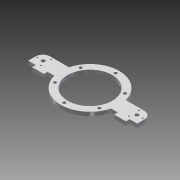
# Autodesk Inventor part: middle plate2
Saved by Autodesk Inventor 2015 (Build 190159000, 159)
## iProperties
Created: 2015-02-28
Part Number: middle plate2
Material: Generic
Document SubType Name: Modeling
Designer: Qiuyang
Density: 1 g/cm^3
Appearance: Default
Author: Qiuyang
Autodesk Inventor part; units mm, degrees
ref_plane "YZ Plane" through (0, 0, 0) normal (1, 0, 0) x (0, 1, 0)
ref_plane "XZ Plane" through (0, 0, 0) normal (0, 1, 0) x (-1, 0, 0)
ref_plane "XY Plane" through (0, 0, 0) normal (0, 0, 1) x (1, 0, 0)
sketch "Sketch4" plane through (0, 0, 0) normal (0, 1, 0) x (-1, 0, 0)
  circle A0 centre (0, 0) radius 38.735
  circle A1 centre (0, 0) radius 50.8
  dimension "d9" = 77.47
  dimension "d10" = 101.6
  constraints: 2 centre point, 2 coincident
  measures "d9" diameter of A0
  measures "d10" diameter of A1
extrude "Extrusion2" add sketch "Sketch4" along normal blind 6.35
sketch "Sketch5" plane through (0, 6.35, 0) normal (0, 1, 0) x (1, 0, 0)
  circle A0 centre (0, -44.45) radius 2.667
  circle A1 centre (38.4948, -22.225) radius 2.667
  circle A2 centre (38.4948, 22.225) radius 2.667
  circle A3 centre (0, 44.45) radius 2.667
  circle A4 centre (-38.4948, 22.225) radius 2.667
  circle A5 centre (-38.4948, -22.225) radius 2.667
  point P0 (0, 0)
  dimension "d13" = 5.334
  dimension "d16" = 360
  constraints: 6 centre point, 13 other
  measures "d13" diameter of A0
extrude "Extrusion3" cut sketch "Sketch5" against normal blind 6.35
sketch "Sketch7" plane through (0, 6.35, 0) normal (0, 1, 0) x (1, 0, 0)
  line L0 (50.8, 12.7) -> (81.788, 12.7)
  line L1 (81.788, 12.7) -> (81.788, -12.7)
  line L2 (81.788, -12.7) -> (50.8, -12.7)
  line L3 (50.8, -12.7) -> (50.8, 12.7)
  line L4 (-50.8, 12.7) -> (-81.788, 12.7)
  line L5 (-81.788, 12.7) -> (-81.788, -12.7)
  line L6 (-81.788, -12.7) -> (-50.8, -12.7)
  line L7 (-50.8, -12.7) -> (-50.8, 12.7)
  point P0 (0, 0)
  dimension "d50" = 30.988
  dimension "d51" = 25.4
  dimension "d52" = 30.988
  constraints: 16 end point, 4 parallel, 2 horizontal, 2 perpendicular, 2 point on line
  measures "d50" distance of L1.end L2.end
  measures "d51" distance of L0.end L1.end
  measures "d52" distance of L6.end L5.end
extrude "Extrusion4" add sketch "Sketch7" against normal blind 6.35
sketch "Sketch8" plane through (0, 6.35, 0) normal (0, 1, 0) x (1, 0, 0)
  line L0 (-123.5202, 12.7) -> (-50.8, 12.7) projected
  line L1 (-60.9386, 12.7) -> (-45.3133, 12.7)
  line L2 (-45.3133, 12.7) -> (-45.3133, -12.7)
  line L3 (-45.3133, -12.7) -> (-60.9386, -12.7)
  line L4 (-60.9386, -12.7) -> (-60.9386, 12.7)
  line L5 (57.1886, 12.7) -> (43.7508, 12.7)
  line L6 (43.7508, 12.7) -> (43.7508, -12.7)
  line L7 (43.7508, -12.7) -> (57.1886, -12.7)
  line L8 (57.1886, -12.7) -> (57.1886, 12.7)
  point P0 (0, 0)
  constraints: 16 end point, 4 parallel, 3 point on line, 2 horizontal, 2 perpendicular
extrude "Extrusion5" add sketch "Sketch8" against normal blind 6.35
sketch "Sketch9" plane through (0, 6.35, 0) normal (0, 1, 0) x (1, 0, 0)
  line L0 (111.76, 12.7) -> (111.76, -12.7) projected
  line L1 (81.788, 12.7) -> (81.788, -12.7) projected
  circle A0 centre (81.788, 0) radius 12.7
  line L2 (-81.788, 12.7) -> (-81.788, -12.7) projected
  circle A1 centre (-81.788, 0) radius 12.7
  point P0 (0, 0)
  point P1 (-111.7602, 0)
  point P2 (-111.76, -12.7)
  constraints: 2 midpoint, 2 vertical alignment, 4 other
extrude "Extrusion6" add sketch "Sketch9" against normal blind 6.35
sketch "Sketch10" plane through (0, 6.35, 0) normal (0, 1, 0) x (1, 0, 0)
  circle A0 centre (81.28, 0) radius 3.175
  circle A1 centre (91.3638, 0) radius 1.27
  circle A2 centre (76.2381, 8.7328) radius 1.27
  circle A3 centre (76.2381, -8.7328) radius 1.27
  circle A4 centre (-81.28, 0) radius 3.175
  circle A5 centre (-91.3638, 0) radius 1.27
  circle A6 centre (-76.2381, -8.7328) radius 1.27
  circle A7 centre (-76.2381, 8.7328) radius 1.27
  point P0 (0, 0)
  dimension "d53" = 6.35
  dimension "d54" = 2.54
  dimension "d57" = 360
  dimension "d59" = 6.35
  dimension "d60" = 2.54
  dimension "d63" = 360
  constraints: 8 centre point, 14 other
  measures "d53" diameter of A0
  measures "d54" diameter of A1
  measures "d59" diameter of A4
  measures "d60" diameter of A5
extrude "Extrusion7" cut sketch "Sketch10" against normal blind 6.35
sketch "Sketch11" plane through (0, 6.35, 0) normal (0, 1, 0) x (1, 0, 0)
  arc A0 (-81.788, 12.7) -> (-81.788, -12.7) centre (-81.788, 0) ccw projected
  line L0 (-94.488, 0) -> (-81.788, 0)
  line L1 (-81.788, 0) -> (-81.788, -12.7)
  line L2 (-81.788, -12.7) -> (-94.488, -12.7)
  line L3 (-94.488, -12.7) -> (-94.488, 0)
  arc A1 (81.788, -12.7) -> (81.788, 12.7) centre (81.788, 0) ccw projected
  line L4 (94.488, 0) -> (81.788, 0)
  line L5 (81.788, 0) -> (81.788, -12.7)
  line L6 (81.788, -12.7) -> (94.488, -12.7)
  line L7 (94.488, -12.7) -> (94.488, 0)
  point P0 (0, 0)
  constraints: 16 end point, 4 parallel, 2 horizontal, 2 perpendicular, 2 point on circle, 1 point on line
extrude "Extrusion8" add sketch "Sketch11" against normal blind 6.35 contours A0 L2 L3 | A1 L7 L6
sketch "Sketch12" plane through (0, 6.35, 0) normal (0, 1, 0) x (1, 0, 0)
  line L0 (-49.1869, -12.7) -> (-94.488, -12.7) projected
  line L1 (-81.28, -12.7) -> (-60.96, -12.7)
  line L2 (-60.96, -12.7) -> (-60.96, -19.05)
  line L3 (-60.96, -19.05) -> (-81.28, -19.05)
  line L4 (-81.28, -19.05) -> (-81.28, -12.7)
  line L5 (94.488, -12.7) -> (49.1869, -12.7) projected
  line L6 (81.28, -12.7) -> (60.96, -12.7)
  line L7 (60.96, -12.7) -> (60.96, -19.05)
  line L8 (60.96, -19.05) -> (81.28, -19.05)
  line L9 (81.28, -19.05) -> (81.28, -12.7)
  point P0 (0, 0)
  dimension "d67" = 20.32
  dimension "d68" = 6.35
  dimension "d69" = 20.32
  constraints: 16 end point, 4 parallel, 3 point on line, 2 horizontal, 2 perpendicular
  measures "d67" distance of L2.end L3.end
  measures "d68" distance of L1.end L2.end
  measures "d69" distance of L8.end L7.end
extrude "Extrusion9" add sketch "Sketch12" against normal blind 6.35
body "Solid2"
